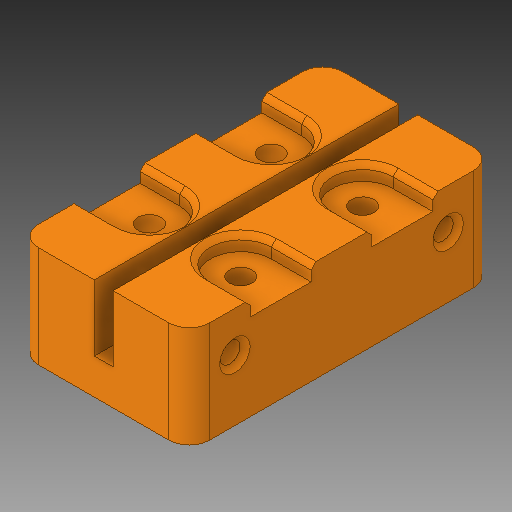
# Autodesk Inventor part: sujetador plancha aluminio
Saved by Autodesk Inventor 2018 (Build 220112000, 112)
## iProperties
Created: 2019-05-18
Part Number: sujetador plancha aluminio
Material: Generic
Document SubType Name: Modeling
Designer: JLVega003
Density: 1 g/cm^3
Appearance: Orange
Author: JLVega003
Autodesk Inventor part; units mm, degrees
ref_plane "YZ Plane" through (0, 0, 0) normal (1, 0, 0) x (0, 1, 0)
ref_plane "XZ Plane" through (0, 0, 0) normal (0, 1, 0) x (-1, 0, 0)
ref_plane "XY Plane" through (0, 0, 0) normal (0, 0, 1) x (1, 0, 0)
sketch "Sketch1" plane through (0, 0, 0) normal (0, 0, 1) x (1, 0, 0)
  line L0 (16.85, 0) -> (-16.85, 0)
  line L1 (-16.85, 0) -> (-16.85, 20)
  line L2 (-16.85, 20) -> (-1.85, 20)
  line L3 (-1.85, 20) -> (-1.85, 7)
  line L4 (-1.85, 7) -> (1.85, 7)
  line L5 (1.85, 7) -> (1.85, 20)
  line L6 (1.85, 20) -> (16.85, 20)
  line L7 (16.85, 20) -> (16.85, 0)
  line L8 (-23.59, 0) -> (23.59, 0) projected
  line L9 (0, -4) -> (0, 24) projected
  point P0 (0, 0)
  point P1 (0, 7)
  point P2 (0, 0)
  dimension "d0" = 33.7
  dimension "d1" = 3.7
  dimension "d2" = 13
  dimension "d3" = 20
  constraints: 16 end point, 6 perpendicular, 4 point on line, 2 midpoint, 1 collinear, 1 horizontal
  measures "d0" distance between parallel lines of L7 L1
  measures "d1" distance between parallel lines of L5 L3
  measures "d2" distance between parallel lines of L6 L4
  measures "d3" distance between parallel lines of L0 L2
extrude "Extrusion1" add sketch "Sketch1" along normal mid plane 60
sketch "Sketch2" plane through (-16.85, 20, 30) normal (0, 1, 0) x (1, 0, 0)
  line L0 (0, 60) -> (0, 0) projected
  line L1 (15, 0) -> (0, 0) projected
  line L2 (15, 60) -> (15, 0) projected
  line L3 (0, 60) -> (15, 60) projected
  line L4 (18.7, 60) -> (18.7, 0) projected
  line L5 (33.7, 0) -> (18.7, 0) projected
  line L6 (33.7, 60) -> (33.7, 0) projected
  line L7 (18.7, 60) -> (33.7, 60) projected
  line L8 (25.85, 42) -> (7.85, 42) construction
  line L9 (7.85, 42) -> (7.85, 18) construction
  line L10 (7.85, 18) -> (25.85, 18) construction
  line L11 (25.85, 18) -> (25.85, 42) construction
  line L12 (25.85, 42) -> (7.85, 18) construction
  line L13 (7.85, 42) -> (25.85, 18) construction
  point P0 (16.85, 30)
  dimension "d6" = 18
  dimension "d7" = 24
  constraints: 12 end point, 4 coincident, 2 midpoint, 2 parallel, 1 horizontal, 1 perpendicular
  measures "d6" distance between parallel lines of L11 L9
  measures "d7" distance between parallel lines of L8 L10
hole "Hole1" at (-9, 20, 12) at (-9, 20, -12) at (9, 20, 12) at (9, 20, -12) direction (0, -1, 0) diameter 4.5 end through all counterbore diameter 12 counterbore depth 3
sketch "Sketch3" plane through (1.85, 20, 30) normal (0, 1, 0) x (1, 0, 0)
  circle A0 centre (-10.85, 18) radius 6 projected
  circle A1 centre (-10.85, 42) radius 6 projected
  line L0 (-18.7, 60) -> (-18.7, 0) projected
  line L1 (-3.7, 0) -> (-18.7, 0) projected
  line L2 (-3.7, 60) -> (-3.7, 0) projected
  line L3 (-18.7, 60) -> (-3.7, 60) projected
  circle A2 centre (7.15, 18) radius 6 projected
  circle A3 centre (7.15, 42) radius 6 projected
  line L4 (0, 60) -> (0, 0) projected
  line L5 (15, 0) -> (0, 0) projected
  line L6 (15, 60) -> (15, 0) projected
  line L7 (0, 60) -> (15, 60) projected
  line L8 (7.15, 12) -> (15, 12)
  line L9 (15, 12) -> (15, 24)
  line L10 (15, 24) -> (7.15, 24)
  line L11 (7.15, 24) -> (7.15, 12)
  line L12 (7.15, 36) -> (15, 36)
  line L13 (15, 36) -> (15, 48)
  line L14 (15, 48) -> (7.15, 48)
  line L15 (7.15, 48) -> (7.15, 36)
  line L16 (-18.7, 36) -> (-10.85, 36)
  line L17 (-10.85, 36) -> (-10.85, 48)
  line L18 (-10.85, 48) -> (-18.7, 48)
  line L19 (-18.7, 48) -> (-18.7, 36)
  line L20 (-18.7, 12) -> (-10.85, 12)
  line L21 (-10.85, 12) -> (-10.85, 24)
  line L22 (-10.85, 24) -> (-18.7, 24)
  line L23 (-18.7, 24) -> (-18.7, 12)
  circle A4 centre (7.15, 18) radius 6 projected
  circle A5 centre (7.15, 42) radius 6 projected
  point P0 (-1.85, 30)
  constraints: 32 end point, 8 parallel, 5 point on line, 4 coincident, 4 horizontal, 4 midpoint, 4 perpendicular, 4 tangent
extrude "Extrusion2" cut sketch "Sketch3" against normal blind 3 contours L21 A0 | A0 L20 L0 L22 | L0 L18 A1 L16 | A1 L17 | A2 L11 | A2 L10 L6 L8 | L12 A3 L14 L6 | L15 A3 picked at (-12.72, 18.7092) picked at (-12.72, 42.7092) picked at (8.397, 19.5637) picked at (8.7137, 43.247)
fillet "Fillet1" radius 4 4 edges at (-16.85, 10, 30) (16.85, 10, 30) (16.85, 10, -30) (-16.85, 10, -30)
chamfer "Chamfer1" distance 1 angle 45 12 edges at (3, 20, -12) (12.925, 20, -18) (12.925, 20, -6) (-12.925, 20, -18) (-3, 20, -12) (-12.925, 20, -6) (-12.925, 20, 6) (-3, 20, 12) (-12.925, 20, 18) (3, 20, 12) (12.925, 20, 6) (12.925, 20, 18)
chamfer "Chamfer2" distance 1 angle 45 4 edges at (-9, 0, 9.75) (9, 0, 9.75) (-9, 0, -14.25) (9, 0, -14.25)
sketch "Sketch4" plane through (16.85, 17, 18) normal (1, 0, 0) x (0, 0, -1)
  line L0 (-3, -5) -> (39, -5) construction
  line L1 (18, -21) -> (18, 7) projected
  line L2 (-1, 3) -> (-8, 3) projected
  point P0 (18, -17)
  point P1 (18, -5)
  dimension "d24" = 42
  dimension "d25" = 8
  constraints: 2 coincident, 2 end point, 1 horizontal, 1 midpoint, 1 point on line
  measures "d24" distance of L0.start L0.end
  measures "d25" distance between parallel lines of L0 L2
hole "Hole2" at (16.85, 12, 21) at (16.85, 12, -21) direction (-1, 0, 0) diameter 4 end through all
chamfer "Chamfer3" distance 1 angle 45 4 edges at (16.85, 12, 23) (16.85, 12, -19) (-16.85, 12, -19) (-16.85, 12, 23)
body "Solid1"
